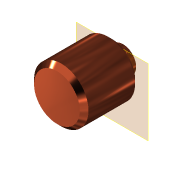
# Autodesk Inventor part: ManualKnob
Saved by Autodesk Inventor 2022 (Build 260153000, 153)
## iProperties
Created: 2023-05-09
Part Number: ManualKnob
Material: Generic
Document SubType Name: Modeling
Designer: UCadmin2
Density: 1 g/cm^3
Appearance: Copper - Polished
Author: UCadmin2
Autodesk Inventor part; units mm, degrees
ref_plane "YZ Plane" through (0, 0, 0) normal (1, 0, 0) x (0, 1, 0)
ref_plane "XZ Plane" through (0, 0, 0) normal (0, 1, 0) x (-1, 0, 0)
ref_plane "XY Plane" through (0, 0, 0) normal (0, 0, 1) x (1, 0, 0)
ref_plane "Work Plane1" through (0, 0, 0) normal (0, 0, 1) x (1, 0, 0)
sketch "Sketch1" plane through (0, 0, 0) normal (0, 0, 1) x (1, 0, 0)
  circle A0 centre (0, 6.35) radius 4 projected
  circle A1 centre (0, 6.35) radius 12.5
  point P0 (0, 0)
  dimension "d0" = 25
  constraints: 1 centre point, 1 coincident
  measures "d0" diameter of A1
extrude "Extrusion1" add sketch "Sketch1" along normal blind 25.4 contours A0 | A1
sketch "Skizze2" plane through (0, 6.35, 0) normal (0, 0, -1) x (-1, 0, 0)
  circle A0 centre (0, 0) radius 11 projected
  circle A1 centre (0, 0) radius 2.9
  point P0 (0, -6.35)
  point P1 (-5.9, 11.95)
  dimension "d3" = 5.8
  constraints: 1 centre point, 1 coincident, 1 other
  measures "d3" diameter of A1
extrude "Extrusion2" cut sketch "Skizze2" against normal blind 20 contours A1
chamfer "Fase1" distance 2 angle 45 2 edges at (-12.5, 6.35, 25.4) (-12.5, 6.35, 0)
sketch "Skizze3" plane through (0, 6.35, 0) normal (0, 0, -1) x (-1, 0, 0)
  circle A0 centre (0, 0) radius 3 projected
  circle A1 centre (0, 0) radius 2.9 projected
  circle A2 centre (0, 0) radius 10.5 projected
  circle A3 centre (0, 0) radius 6
  point P0 (0, -6.35)
  dimension "d9" = 12
  constraints: 1 centre point, 1 coincident
  measures "d9" diameter of A3
extrude "Extrusion3" add sketch "Skizze3" along normal blind 5 contours A3
sketch "Skizze4" plane through (0, 0, 0) normal (1, 0, 0) x (0, 1, 0)
  circle A0 centre (6.1822, -2.4807) radius 1.4
  point P0 (0, 0)
  dimension "d12" = 2.8
  constraints: 1 centre point
  measures "d12" diameter of A0
extrude "Extrusion4" cut sketch "Skizze4" against normal through all
pattern_circular "Runde Anordnung1" count 3 over 360 about axis through (0, 6.35, 0) along (0, 0, -1) of "Extrusion4"
body "Solid1"
